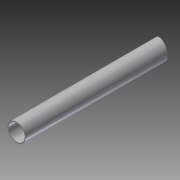
# Autodesk Inventor part: GE-13018-01
Saved by Autodesk Inventor 2013 (Build 170138000, 138)
## iProperties
Created: 2013-01-06
Part Number: GE-13018-01
Material: Steel
Document SubType Name: Modeling
Designer: Phillip
Density: 1 g/cm^3
Author: Phillip
Autodesk Inventor part; units mm, degrees
ref_plane "YZ Plane" through (0, 0, 0) normal (1, 0, 0) x (0, 1, 0)
ref_plane "XY Plane" through (0, 0, 0) normal (0, 0, 1) x (1, 0, 0)
sketch "Sketch1" plane through (0, 0, 0) normal (0, 0, 1) x (1, 0, 0)
  circle A0 centre (0, 0) radius 16.891
  circle A1 centre (0, 0) radius 19.05
  dimension "d0" = 38.1
  dimension "d2" = 33.782
  constraints: 2 centre point, 2 coincident
  measures "d0" diameter of A1
  measures "d2" diameter of A0
extrude "Extrusion1" add sketch "Sketch1" against normal blind 304.8
ref_plane "Work Plane1" through (0, 19.05, 0) normal (0, 1, 0) x (-1, 0, 0)
sketch "Sketch2" plane through (0, 19.05, 0) normal (0, 1, 0) x (-1, 0, 0)
  line L0 (19.05, 0) -> (19.05, -304.8) projected
  line L1 (-19.05, -304.8) -> (19.05, -304.8) projected
  line L2 (19.05, -304.8) -> (-19.05, -294.5911)
  line L3 (-19.05, 0) -> (-19.05, -304.8) projected
  point P0 (0, 0)
  dimension "d5" = 15
  constraints: 2 end point, 1 point on line
  measures "d5" angle of L1 L2
extrude "Extrusion2" cut sketch "Sketch2" against normal blind 50.8
sketch "Sketch3" plane through (0, 0, 0) normal (0, 1, 0) x (-1, 0, 0)
  line L0 (19.05, 0) -> (19.05, -304.8) projected
  point P0 (0, 0)
body "Solid1"
